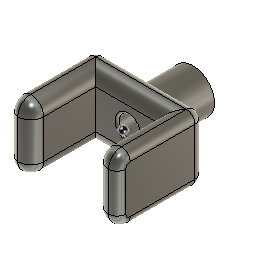
key_turner_autodoorlock v3 (Autodesk Fusion 360 design; units mm, degrees)
Autodesk Fusion 360 part; units mm, degrees
sketch "Sketch1" plane through (0, 0, 0) normal (0, 0, 1) x (1, 0, 0)
  line L0 (-40, 15) -> (-15, 15)
  line L1 (-15, 15) -> (-15, 10)
  line L2 (-15, 10) -> (-40, 10)
  line L3 (-40, 10) -> (-40, 15)
  dimension "d1" = 25
  dimension "d2" = 5
  constraint horizontal L0
  constraint vertical L1
  constraint horizontal L2
  constraint vertical L3
  measures "d1" distance of L0.start L0.end
  measures "d2" distance of L0.start L2.end
extrude "Extrude1" add sketch "Sketch1" along normal blind 15
sketch "Sketch2" plane through (0, 10, 0) normal (0, -1, 0) x (1, 0, 0)
  line L0 (-40, 0) -> (-15, 0)
  line L1 (-15, 0) -> (-15, 15)
  line L2 (-15, 15) -> (-40, 15)
  line L3 (-40, 15) -> (-40, 0)
  line L4 (-40, 15) -> (-35, 15)
  line L5 (-35, 15) -> (-35, 0)
  line L6 (-35, 0) -> (-40, 0)
  line L7 (-40, 0) -> (-40, 15)
  line L8 (-15, 15) -> (-20, 15)
  line L9 (-20, 15) -> (-20, 0)
  line L10 (-20, 0) -> (-15, 0)
  line L11 (-15, 0) -> (-15, 15)
  dimension "d5" = 5
  dimension "d6" = 5
  dimension "d7" = 15
  constraint horizontal L4
  constraint vertical L5
  constraint horizontal L6
  constraint vertical L7
  constraint coincident L2.end L3.start
  constraint horizontal L8
  constraint vertical L9
  constraint horizontal L10
  constraint vertical L11
  constraint coincident L1.end L2.start
  measures "d5" distance of L2.end L4.end
  measures "d6" distance of L1.end L8.end
  measures "d7" distance of L1.end L0.end
extrude "Extrude2" add sketch "Sketch2" along normal blind 15 contours L0 L2 L3 L4 L5 L6 L7
sketch "Sketch3" plane through (0, 10, 0) normal (0, -1, 0) x (1, 0, 0)
  line L0 (-35, 15) -> (-35, 0)
  line L1 (-35, 0) -> (-15, 0)
  line L2 (-15, 0) -> (-15, 15)
  line L3 (-15, 15) -> (-35, 15)
  line L4 (-15, 15) -> (-20, 15)
  line L5 (-20, 15) -> (-20, 0)
  line L6 (-20, 0) -> (-15, 0)
  line L7 (-15, 0) -> (-15, 15)
  dimension "d10" = 5
  dimension "d11" = 15
  constraint horizontal L4
  constraint vertical L5
  constraint horizontal L6
  constraint vertical L7
  constraint coincident L2.end L3.start
  measures "d10" distance of L2.end L4.end
  measures "d11" distance of L2.end L1.end
extrude "Extrude3" add sketch "Sketch3" along normal blind 15 contours L1 L2 L3 L4 L5 L6 L7
fillet "Fillet1" radius 3 3 edges at (-27.5, 10, 15) (-35, 2.5, 15) (-20, 2.5, 15)
fillet "Fillet2" radius 3 6 edges at (-20, -5, 6) (-19.1213, -5, 14.1213) (-16, -5, 15) (-35, -5, 6) (-35.8787, -5, 14.1213) (-39, -5, 15)
fillet "Fillet3" radius 3 7 edges at (-27.5, 10, 0) (-20, 4, 0) (-19.1213, -4.1213, 0) (-16, -5, 0) (-35, 4, 0) (-35.8787, -4.1213, 0) (-39, -5, 0)
fillet "Fillet4" radius 2 5 edges at (-40, 6.5, 15) (-40, -4.1213, 14.1213) (-40, -5, 7.5) (-40, -4.1213, 0.8787) (-40, 6.5, 0)
fillet "Fillet5" radius 2 10 edges at (-15, 6.5, 15) (-15, -4.1213, 14.1213) (-15, -5, 7.5) (-15, -4.1213, 0.8787) (-15, 6.5, 0) (-26.5, 15, 15) (-39.4142, 15, 14.4142) (-40, 15, 7.5) (-39.4142, 15, 0.5858) (-26.5, 15, 0)
fillet "Fillet6" radius 2 3 edges at (-15.5858, 14.4142, 0.5858) (-15, 15, 7.5) (-15.5858, 14.4142, 14.4142)
sketch "Sketch4" plane through (0, 15, 0) normal (0, 1, 0) x (-1, 0, 0)
  line L0 (17, 13) -> (17, 2)
  line L1 (17, 2) -> (38, 2)
  line L2 (38, 2) -> (38, 13)
  line L3 (38, 13) -> (17, 13)
  circle A0 centre (27.5, 7.5) radius 5
  circle A1 centre (27.5, 7.5) radius 2.5
  point P0 (27.5, 7.5)
  dimension "d26" = 10
  dimension "d27" = 5
  constraint coincident P0 A0.centre
  measures "d26" diameter of A0
  measures "d27" diameter of A1
extrude "Extrude4" add sketch "Sketch4" along normal blind 10 contours A0
fillet "Fillet7" radius 1 1 edges at (-22.8384, 15, 9.3081)
hole "Hole1" at (-27.5, 15, 7.5) direction (0, -1, 0) diameter 5 depth 5.1 tip angle 118
fillet "Fillet8" radius 0.5 1 edges at (-28.404, 10, 5.1692)
sketch "Sketch5" plane through (0, 0, 0) normal (0, 0, 1) x (1, 0, 0)
